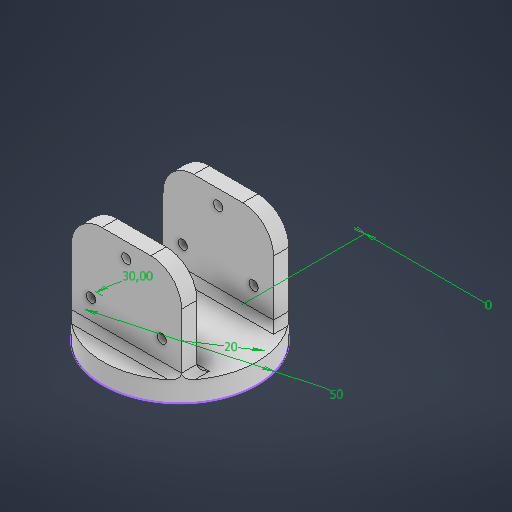
# Autodesk Inventor part: rotacniZaklad
Saved by Autodesk Inventor 2026 (Build 300175000, 175)
## iProperties
Created: 2025-04-11
Part Number: rotacniZaklad
Material: Generic
Document SubType Name: Modeling
Designer: vitgr
Density: 1 g/cm^3
Appearance: Default
Author: vitgr
Autodesk Inventor part; units mm, degrees
ref_plane "YZ Plane" through (0, 0, 0) normal (1, 0, 0) x (0, 1, 0)
ref_plane "XZ Plane" through (0, 0, 0) normal (0, 1, 0) x (-1, 0, 0)
ref_plane "XY Plane" through (0, 0, 0) normal (0, 0, 1) x (1, 0, 0)
sketch "Sketch1" plane through (0, 0, 0) normal (0, 1, 0) x (-1, 0, 0)
  line L0 (17.3205, -10) -> (21.6506, -12.5)
  line L1 (0, 0) -> (25, 0) construction
  line L2 (17.3205, 10) -> (21.6506, 12.5)
  line L3 (-17.3205, -10) -> (-21.6506, -12.5)
  line L4 (-17.3205, 10) -> (-21.6506, 12.5)
  arc A0 (17.3205, 10) -> (-17.3205, 10) centre (0, 0) ccw
  arc A1 (-17.3205, -10) -> (17.3205, -10) centre (0, 0) ccw
  arc A2 (21.6506, 12.5) -> (-21.6506, 12.5) centre (0, 0) ccw
  arc A3 (-21.6506, -12.5) -> (21.6506, -12.5) centre (0, 0) ccw
  circle A4 centre (0, 0) radius 25
  point P0 (0, -20)
  point P1 (0, -20)
  dimension "d13" = 50
  dimension "d4" = 30
  dimension "d10" = 0
  dimension "d11" = 20
  constraints: 10 end point, 10 point on circle, 4 centre point, 2 coincident, 1 horizontal, 1 symmetric about line, 3 other
  measures "d4" angle of L0 L1
  measures "d10" distance of point (0, -20) point (0, -20)
  measures "d11" radius of A1
sketch "Sketch2" plane through (0, 0, 0) normal (0, 1, 0) x (-1, 0, 0)
  circle A0 centre (0, 0) radius 25
  dimension "d14" = 50
  constraints: 1 centre point, 1 coincident
  measures "d14" diameter of A0
extrude "Extrusion1" add sketch "Sketch2" along normal blind 6.5
sketch "Sketch3" plane through (0, 6.5, 0) normal (0, 1, 0) x (1, 0, 0)
  circle A0 centre (0, 0) radius 25
  circle A1 centre (0, 0) radius 25
  line L0 (-17.9368, 12.4147) -> (-17.9368, 17.4147)
  line L1 (-17.9368, 17.4147) -> (17.9368, 17.4147)
  line L2 (-25, 0) -> (25, 0)
  line L3 (17.9368, 17.4147) -> (17.9368, 12.4147)
  line L4 (17.9368, 12.4147) -> (-17.9368, 12.4147)
  line L5 (-17.9368, -12.4147) -> (-17.9368, -17.4147)
  line L6 (-17.9368, -17.4147) -> (17.9368, -17.4147)
  line L7 (17.9368, -17.4147) -> (17.9368, -12.4147)
  line L8 (17.9368, -12.4147) -> (-17.9368, -12.4147)
  dimension "d23" = 35.8735
  dimension "d24" = 5
  constraints: 18 end point, 4 point on circle, 4 symmetric about line, 2 centre point, 2 coincident, 2 horizontal, 2 perpendicular, 1 parallel
  measures "d23" distance of L0.end L1.end
  measures "d24" distance of L1.end L3.end
extrude "Extrusion3" add sketch "Sketch3" along normal blind 30 contours L3 L4 L0 L1 | L6 L5 L8 L7
fillet "Fillet1" radius 2 8 edges at (0, 6.5, 12.4147) (17.9368, 6.5, 14.9147) (17.9368, 6.5, -14.9147) (0, 6.5, -12.4147) (0, 6.5, 17.4147) (-17.9368, 6.5, 14.9147) (-17.9368, 6.5, -14.9147) (0, 6.5, -17.4147)
fillet "Fillet2" radius 10 4 edges at (17.9368, 36.5, 14.9147) (-17.9368, 36.5, 14.9147) (-17.9368, 36.5, -14.9147) (17.9368, 36.5, -14.9147)
sketch "Sketch4" plane through (-17.9368, 8.5, 17.4147) normal (0, 0, 1) x (1, 0, 0)
  circle A0 centre (17.9368, 23.2043) radius 1.5
  circle A1 centre (6.45, 6.5) radius 1.5
  circle A2 centre (29.45, 6.5) radius 1.5
  line L0 (42.9368, -8.5) -> (-7.0632, -8.5) projected
  line L1 (0, 0) -> (0, 18) projected
  line L2 (35.8735, 0) -> (35.8735, 18) projected
  point P0 (17.9368, -8.5)
  dimension "d29" = 3
  dimension "d30" = 3
  dimension "d31" = 3
  dimension "d32" = 15
  dimension "d33" = 15
  dimension "d34" = 20
  dimension "d35" = 6.45
  dimension "d36" = 6.4235
  constraints: 3 centre point
  measures "d29" diameter of A0
  measures "d30" diameter of A2
  measures "d31" diameter of A1
  measures "d32" distance from line of L0 A1.centre
  measures "d33" distance from line of L0 A2.centre
  measures "d35" distance from line of L1 A1.centre
  measures "d36" distance from line of L2 A2.centre
extrude "Extrusion4" cut sketch "Sketch4" against normal blind 82
sketch "Sketch5" plane through (0, 0, 0) normal (0, -1, 0) x (1, 0, 0)
  circle A0 centre (0, 0) radius 2.9
  dimension "d39" = 5.8
  constraints: 1 centre point, 1 coincident
  measures "d39" diameter of A0
extrude "Extrusion5" cut sketch "Sketch5" against normal blind 3.6
body "Solid1"
